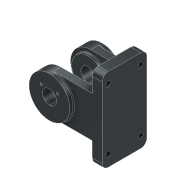
# Autodesk Inventor part: Вилка
Saved by Autodesk Inventor 2021 (Build 250183000, 183)
## iProperties
Created: 2022-05-01
Part Number: Вилка
Material: Iron, Cast
Document SubType Name: Modeling
Designer: DuctopwH
Density: 7.15 g/cm^3
Appearance: Iron Gray
Author: DuctopwH
Autodesk Inventor part; units mm, degrees
ref_plane "YZ Plane" through (0, 0, 0) normal (1, 0, 0) x (0, 1, 0)
ref_plane "XZ Plane" through (0, 0, 0) normal (0, 1, 0) x (-1, 0, 0)
ref_plane "XY Plane" through (0, 0, 0) normal (0, 0, 1) x (1, 0, 0)
sketch "Sketch1" plane through (0, 0, 0) normal (0, 0, 1) x (1, 0, 0)
  line L0 (13, -102) -> (-13, -102)
  line L1 (-13, -102) -> (-13, 102)
  line L2 (-13, 102) -> (13, 102)
  line L3 (13, 102) -> (13, -102)
  line L4 (13, -102) -> (-13, 102) construction
  line L5 (-13, -102) -> (13, 102) construction
  point P0 (0, 0)
  dimension "d0" = 26
  dimension "d1" = 204
  constraints: 12 end point, 2 midpoint, 2 parallel, 1 horizontal, 1 perpendicular
  measures "d0" distance between parallel lines of L3 L1
  measures "d1" distance between parallel lines of L0 L2
extrude "Extrusion1" add sketch "Sketch1" along normal mid plane 110
sketch "Sketch2" plane through (0, 0, 55) normal (0, 0, 1) x (1, 0, 0)
  line L0 (0, 0) -> (-107, 0)
  circle A0 centre (-107, 0) radius 17.5
  circle A1 centre (-107, 0) radius 50
  line L1 (-107, 50) -> (-13, 50)
  line L2 (-13, 102) -> (-13, -102) projected
  line L3 (-107, -50) -> (-13, -50)
  line L4 (13, -102) -> (13, 102) projected
  point P0 (-13, -50)
  dimension "d5" = 100
  dimension "d4" = 35
  dimension "d6" = 120
  constraints: 6 end point, 3 horizontal, 2 coincident, 2 symmetric about line, 1 centre point, 1 point on line, 3 other
  measures "d4" diameter of A0
  measures "d6" distance from line of L4 L0.end
extrude "Extrusion2" add sketch "Sketch2" against normal blind 18
sketch "Sketch3" plane through (0, 0, 55) normal (0, 0, 1) x (1, 0, 0)
  circle A0 centre (-107, 0) radius 17.5 projected
  arc A1 (-107, 50) -> (-107, -50) centre (-107, 0) ccw projected
  circle A2 centre (-107, 0) radius 50
  point P0 (0, 0)
  point P1 (-107, -50)
  constraints: 1 centre point, 1 coincident, 1 concentric
extrude "Extrusion3" add sketch "Sketch3" along normal blind 10
sketch "Sketch4" plane through (0, 0, 37) normal (0, 0, -1) x (-1, 0, 0)
  circle A0 centre (107, 0) radius 17.5 projected
  circle A1 centre (107, 0) radius 40
  point P0 (0, 0)
  dimension "d11" = 80
  constraints: 1 centre point, 1 coincident
  measures "d11" diameter of A1
extrude "Extrusion4" add sketch "Sketch4" along normal blind 7
mirror "Mirror1" about plane through (0, 0, 0) normal (0, 0, 1) of "Extrusion2", "Extrusion3", "Extrusion4"
sketch "Sketch5" plane through (-13, -102, -55) normal (-1, 0, 0) x (0, 0, 1)
  line L0 (110, 204) -> (0, 204) projected
  line L1 (55, 204) -> (55, 0)
  line L2 (0, 0) -> (110, 0) projected
  line L3 (55, 102) -> (110, 102)
  circle A0 centre (95, 177) radius 6.5
  circle A1 centre (15, 177) radius 6.5
  circle A2 centre (95, 27) radius 6.5
  circle A3 centre (15, 27) radius 6.5
  dimension "d14" = 13
  dimension "d15" = 80
  dimension "d16" = 150
  constraints: 4 centre point, 4 end point, 3 symmetric about line, 2 midpoint, 1 horizontal, 3 other
  measures "d14" diameter of A1
  measures "d15" distance of A0.centre A1.centre
  measures "d16" distance of A3.centre A1.centre
extrude "Extrusion5" cut sketch "Sketch5" against normal through all both and the other way through all
sketch "Sketch6" plane through (-107, 0, 65) normal (0, 0, 1) x (1, 0, 0)
  circle A0 centre (0, 0) radius 17.5 projected
  line L0 (0, 0) -> (0, 17)
  line L1 (0, 17) -> (20, 17) construction
  line L2 (0, 17) -> (-20, 17) construction
  point P0 (107, 0)
  dimension "d19" = 17
  dimension "d20" = 40
  constraints: 6 end point, 2 coincident, 1 collinear, 1 horizontal, 1 perpendicular, 1 vertical
  measures "d19" distance from line of L0.start L2
  measures "d20" distance of point (20, 17) L2.end
hole "Hole1" at (-87, 17, 65) at (-127, 17, 65) direction (0, 0, -1) diameter 4.917 depth 26 tip angle 118 thread size "M6x1" class "6H" standard "ANSI Metric M Profile"
chamfer "Chamfer1" distance 0.5 angle 45 2 edges at (-87, 19.4585, 65) (-127, 19.4585, 65)
sketch "Sketch7" plane through (0, 0, 0) normal (0, 1, 0) x (-1, 0, 0)
  line L0 (172, -75) -> (142, -75)
  line L1 (142, -75) -> (142, -55)
  line L2 (142, -55) -> (172, -55)
  line L3 (172, -55) -> (172, -75)
  line L4 (157, -65) -> (57, -65) projected
  line L5 (172, -75) -> (142, -55) construction
  line L6 (142, -75) -> (172, -55) construction
  line L7 (157, -37) -> (157, -65) projected
  point P0 (0, 0)
  dimension "d31" = 15
  dimension "d32" = 10
  constraints: 12 end point, 2 midpoint, 2 parallel, 1 horizontal, 1 perpendicular
  measures "d31" distance between parallel lines of L1 L7
  measures "d32" distance between parallel lines of L2 L4
extrude "Extrusion6" cut sketch "Sketch7" against normal through all both and the other way through all
fillet "Fillet1" radius 15 4 edges at (0, 102, -55) (0, 102, 55) (0, -102, -55) (0, -102, 55)
fillet "Fillet2" radius 2 20 edges at (-13, 97.6066, 50.6066) (-13, 68.5, 55) (-13, 97.6066, -50.6066) (-13, 68.5, -55) (-13, 102, 0) (-13, -97.6066, 50.6066) (-13, -68.5, 55) (-13, -97.6066, -50.6066) (-13, -68.5, -55) (-13, -102, 0) (-13, -50, 46) (-13, -50, -46) (-13, 50, -46) (-13, 50, 46) (-13, 0, -37) (-13, 0, 37) (-57, 0, -55) (-57, 0, 55) (-67, 0, -37) (-67, 0, 37)
body "Solid1"
